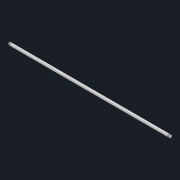
# Autodesk Inventor part: BarraEnLPreDoblado
Saved by Autodesk Inventor 2021 (Build 250183000, 183)
## iProperties
Created: 2021-05-11
Part Number: BarraEnLPreDoblado
Material: Generic
Document SubType Name: Modeling
Designer: GABRIEL LOL
Density: 1 g/cm^3
Appearance: Default
Author: GABRIEL LOL
Autodesk Inventor part; units mm, degrees
ref_plane "YZ Plane" through (0, 0, 0) normal (1, 0, 0) x (0, 1, 0)
ref_plane "XZ Plane" through (0, 0, 0) normal (0, 1, 0) x (-1, 0, 0)
ref_plane "XY Plane" through (0, 0, 0) normal (0, 0, 1) x (1, 0, 0)
sketch "Sketch1" plane through (0, 0, 0) normal (1, 0, 0) x (0, 1, 0)
  circle A0 centre (0, 0) radius 1.5
  dimension "d0" = 3
  constraints: 1 centre point, 1 coincident
  measures "d0" diameter of A0
extrude "Extrusion1" add sketch "Sketch1" along normal blind 180.925
thread "Thread1" size "M3x0.5" class "6g" standard "ANSI Metric M Profile" length 2.5
thread "Thread2" size "M3x0.5" class "6g" standard "ANSI Metric M Profile" length 2.5
body "Solid1"
